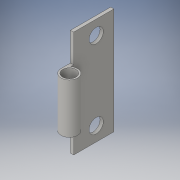
# Autodesk Inventor part: Hinge Wall 1
Saved by Autodesk Inventor 2016 (Build 200138000, 138)
## iProperties
Created: 2016-04-01
Part Number: Hinge Wall 1
Material: Generic
Document SubType Name: Modeling
Designer: amycroft3
Density: 1 g/cm^3
Appearance: Default
Author: amycroft3
Autodesk Inventor part; units mm, degrees
ref_plane "YZ Plane" through (0, 0, 0) normal (1, 0, 0) x (0, 1, 0)
ref_plane "XZ Plane" through (0, 0, 0) normal (0, 1, 0) x (-1, 0, 0)
ref_plane "XY Plane" through (0, 0, 0) normal (0, 0, 1) x (1, 0, 0)
sketch "Sketch1" plane through (0, 0, 0) normal (0, 1, 0) x (-1, 0, 0)
  circle A0 centre (0, 0) radius 2.3876
  arc A1 (2.9591, 0) -> (1.8161, -2.3362) centre (0, 0) ccw
  line L0 (2.9591, 0) -> (2.3876, 0)
  line L1 (1.8161, -2.3362) -> (1.8161, -17.78)
  line L2 (1.8161, -17.78) -> (2.9591, -17.78)
  line L3 (2.9591, -17.78) -> (2.9591, 0)
  dimension "d0" = 4.7752
  dimension "d1" = 5.9182
  dimension "d2" = 17.78
  dimension "d3" = 1.143
  constraints: 8 end point, 2 coincident, 2 parallel, 2 point on circle, 1 centre point, 1 horizontal, 1 horizontal alignment, 1 perpendicular, 1 tangent, 2 other
  measures "d1" diameter of A1
  measures "d2" distance of L2.end L0.start
  measures "d3" distance of L1.end L2.end
extrude "Extrusion1" add sketch "Sketch1" along normal blind 38.1
sketch "Sketch2" plane through (0, 38.1, 0) normal (0, 1, 0) x (1, 0, 0)
  line L0 (-4.1424, -3.452) -> (4.5842, -3.452)
  line L1 (4.5842, -3.452) -> (4.5842, 3.3967)
  line L2 (4.5842, 3.3967) -> (-4.1424, 3.3967)
  line L3 (-4.1424, 3.3967) -> (-4.1424, -3.452)
  point P0 (0, 0)
  dimension "d6" = 8.7266
  dimension "d7" = 6.8487
  dimension "d8" = 4.5842
  dimension "d9" = 3.3967
  constraints: 8 end point, 2 parallel, 1 horizontal, 1 perpendicular
  measures "d6" distance between parallel lines of L1 L3
  measures "d7" distance between parallel lines of L0 L2
  measures "d8" distance from line of point (0, 0) L1
  measures "d9" distance from line of point (0, 0) L2
sketch "Sketch3" plane through (0, 0, 0) normal (0, -1, 0) x (1, 0, 0)
  line L0 (-4.1424, -3.3967) -> (-4.1424, 3.452) projected
  line L1 (-4.1424, 3.452) -> (4.5842, 3.452) projected
  line L2 (4.5842, 3.452) -> (4.5842, -3.3967) projected
  line L3 (4.5842, -3.3967) -> (-4.1424, -3.3967) projected
  point P0 (0, 0)
extrude "Extrusion2" cut sketch "Sketch3" against normal blind 10.16
extrude "Extrusion3" cut sketch "Sketch2" against normal blind 10.16
sketch "Sketch4" plane through (-1.8161, 0, -3.7778) normal (1, 0, 0) x (0, 0, -1)
  circle A0 centre (7.6522, 5.08) radius 2.54
  circle A1 centre (7.6522, 33.02) radius 2.54
  line L0 (14.0022, 0) -> (14.0022, 38.1)
  line L1 (0, 0) -> (14.0022, 0)
  line L2 (0, 38.1) -> (14.0022, 38.1)
  line L3 (14.0022, 0) -> (14.0022, 38.1) projected
  line L4 (-0.381, 38.1) -> (14.0022, 38.1) projected
  line L5 (-0.381, 0) -> (14.0022, 0) projected
  point P0 (-2.3362, 0)
  dimension "d17" = 6.35
  dimension "d16" = 5.08
  dimension "d15" = 5.08
  dimension "d14" = 5.08
  dimension "d21" = 14.0022
  dimension "d22" = 14.0022
  dimension "d23" = 16.3385
  dimension "d24" = 38.1
  constraints: 6 end point, 3 collinear, 2 centre point, 1 equal radius, 1 horizontal, 1 vertical alignment
  measures "d17" distance from line of A0.centre L0
  measures "d16" distance from line of A0.centre L1
  measures "d15" diameter of A0
  measures "d14" distance from line of A1.centre L2
  measures "d21" distance from line of L2.start L3
  measures "d22" distance from line of L1.start L3
  measures "d23" distance from line of point (-2.336, 0) L3
  measures "d24" distance from line of point (-2.336, 0) L4
extrude "Extrusion4" cut sketch "Sketch4" against normal up to next
equation "\"d14\" = d16"
body "Solid1"
